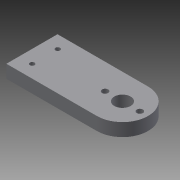
# Autodesk Inventor part: Motor_Mount_Face
Saved by Autodesk Inventor 2016 (Build 200138000, 138)
## iProperties
Created: 2016-04-07
Part Number: Motor_Mount_Face
Material: Generic
Document SubType Name: Modeling
Designer: Ethan
Density: 1 g/cm^3
Appearance: Default
Author: Ethan
Autodesk Inventor part; units mm, degrees
ref_plane "YZ Plane" through (0, 0, 0) normal (1, 0, 0) x (0, 1, 0)
ref_plane "XZ Plane" through (0, 0, 0) normal (0, 1, 0) x (-1, 0, 0)
ref_plane "XY Plane" through (0, 0, 0) normal (0, 0, 1) x (1, 0, 0)
sketch "Sketch1" plane through (0, 0, 0) normal (0, 1, 0) x (-1, 0, 0)
  line L0 (19.05, 12.5) -> (-25.2, 12.5)
  line L1 (-25.2, -12.5) -> (19.05, -12.5)
  line L2 (19.05, -12.5) -> (19.05, 12.5)
  arc A0 (-25.2, 12.5) -> (-25.2, -12.5) centre (-25.2, 0) ccw
  circle A1 centre (12.7, 6.25) radius 1.1303
  circle A2 centre (12.7, -6.25) radius 1.1303
  circle A3 centre (-25.2, 0) radius 4
  circle A4 centre (-16.7, 0) radius 1.5
  circle A5 centre (-33.7, 0) radius 1.5
  point P0 (0, 0)
  dimension "d0" = 44.25
  dimension "d1" = 25
  dimension "d3" = 2.2606
  dimension "d4" = 6.25
  dimension "d5" = 6.35
  dimension "d6" = 19.05
  dimension "d7" = 8
  dimension "d8" = 3
  dimension "d9" = 8.5
  dimension "d10" = 3
  dimension "d11" = 8.5
  constraints: 6 centre point, 6 end point, 2 point on circle, 1 coincident, 1 horizontal, 1 parallel
  measures "d0" distance of L0.start L0.end
  measures "d1" distance of L1.end L0.start
  measures "d3" diameter of A1
  measures "d4" vertical distance of A1.centre point (0, 0)
  measures "d5" distance from line of L2 A1.centre
  measures "d6" distance from line of point (0, 0) L2
  measures "d7" diameter of A3
  measures "d8" diameter of A4
  measures "d9" distance of A4.centre A0.centre
  measures "d10" diameter of A5
  measures "d11" distance of A0.centre A5.centre
extrude "Extrusion1" add sketch "Sketch1" along normal blind 6.35
body "Solid1"
